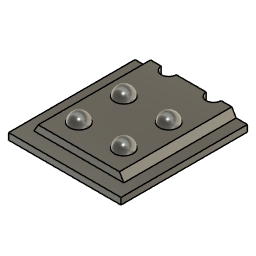
Rivets_Single riveted, single strap butt joint_Model (Autodesk Fusion 360 design; units mm, degrees)
Autodesk Fusion 360 part; units mm, degrees
note: some values were not read from the file. Set by a fixed rule: which sketch regions a step uses.
sketch "Sketch1" plane through (0, 0, 0) normal (0, 1, 0) x (1, 0, 0)
  line L0 (0, 0) -> (-60, 0)
  line L1 (-60, 0) -> (-60, 7)
  line L2 (-60, 7) -> (60, 7)
  line L3 (60, 7) -> (60, 0)
  line L4 (60, 0) -> (0, 0)
  line L5 (0, 0) -> (-48, 0)
  line L6 (0, 0) -> (48, 0)
  line L7 (0, 0) -> (0, -8)
  line L8 (0, -8) -> (-43.3812, -8)
  line L9 (-43.3812, -8) -> (0, -8)
  line L10 (0, -8) -> (43.3812, -8)
  line L11 (48, 0) -> (43.3812, -8)
  line L12 (48, 0) -> (78, 0) construction
  line L13 (-48, 0) -> (-43.3812, -8)
  line L14 (-48, 0) -> (-6.4505, 0) construction
  dimension "d1" = 60
  dimension "d2" = 7
  dimension "d3" = 120
  dimension "d4" = 7
  dimension "d5" = 48
  dimension "d6" = 48
  dimension "d7" = 8
  dimension "d9" = 120
  dimension "d11" = 60
  constraint coincident L0.start L4.end
  constraint horizontal L0
  constraint perpendicular L0 L1
  constraint perpendicular L1 L2
  constraint perpendicular L2 L3
  constraint perpendicular L3 L5
  constraint parallel L4 L6
  constraint perpendicular L6 L7
  constraint perpendicular L7 L8
  constraint perpendicular L7 L10
  constraint horizontal L12
  constraint horizontal L14
  measures "d1" distance of L0.start L0.end
  measures "d2" distance of L0.end L1.end
  measures "d3" distance of L1.end L2.end
  measures "d4" distance of L2.end L3.end
  measures "d5" distance of L0.start L5.end
  measures "d6" distance of L0.start L6.end
  measures "d7" distance of L0.start L7.end
  measures "d9" angle of L11 L12
  measures "d11" angle of L13 L14
extrude "Extrude1" add sketch "Sketch1" along normal mid plane 120 makes body 1
sketch "Sketch2" plane through (0, -60, 0) normal (0, -1, 0) x (1, 0, 0)
  line L0 (-48, 0) -> (-60, 0)
  line L1 (-60, 0) -> (-60, -7)
  line L2 (-60, -7) -> (60, -7)
  line L3 (60, -7) -> (60, 0)
  line L4 (60, 0) -> (48, 0)
  line L5 (48, 0) -> (43.3812, 8)
  line L6 (43.3812, 8) -> (-43.3812, 8)
  line L7 (-43.3812, 8) -> (-48, 0)
  line L8 (-48, 0) -> (48, 0)
  line L9 (48, 0) -> (60, 0)
  line L10 (60, 0) -> (60, -7)
  line L11 (60, -7) -> (-60, -7)
  line L12 (-60, -7) -> (-60, 0)
  line L13 (-60, 0) -> (-48, 0)
  constraint coincident L0.start L7.end
  constraint coincident L4.end L5.start
  constraint coincident L3.end L4.start
  constraint coincident L2.end L3.start
  constraint coincident L1.end L2.start
  constraint coincident L0.end L1.start
extrude "Extrude2" add sketch "Sketch2" along normal blind 15 contours L0 L1 L2 L3 L4 L8 L9 L10 L11 L12 L13 bodies 1
sketch "Sketch3" plane through (0, 0, 8) normal (0, 0, 1) x (-1, 0, 0)
  line L0 (-43.3812, 60) -> (-43.3812, -60)
  line L1 (-43.3812, -60) -> (43.3812, -60)
  line L2 (43.3812, -60) -> (43.3812, 60)
  line L3 (43.3812, 60) -> (-43.3812, 60)
  line L4 (0, -60) -> (0, 60)
  line L5 (0, -60) -> (24, -60)
  line L6 (24, 60) -> (-24, 60)
  circle A0 centre (-24, -60) radius 8
  circle A1 centre (24, -60) radius 8
  circle A2 centre (24, -12) radius 8
  circle A3 centre (24, 36) radius 8
  circle A4 centre (-24, -12) radius 8
  circle A5 centre (-24, 36) radius 8
  dimension "d16" = 24
  dimension "d17" = 24
  dimension "d18" = 48
  dimension "d19" = 16
  dimension "d20" = 16
  dimension "d21" = 48
  dimension "d22" = 16
  dimension "d23" = 48
  dimension "d24" = 16
  dimension "d25" = 48
  dimension "d26" = 16
  dimension "d27" = 48
  dimension "d28" = 16
  constraint midpoint L1 L4.start
  constraint midpoint L3 L4.end
  constraint perpendicular L4 L5
  constraint coincident L3 L6.start
  constraint perpendicular L4 L6
  constraint coincident L5.end A1.centre
  measures "d16" distance of L4.start A0.centre
  measures "d17" distance of L4.start L5.end
  measures "d18" distance of L6.start L6.end
  measures "d19" diameter of A0
  measures "d20" diameter of A1
  measures "d21" distance of L5.end A2.centre
  measures "d22" diameter of A2
  measures "d23" distance of A2.centre A3.centre
  measures "d24" diameter of A3
  measures "d25" distance of A0.centre A4.centre
  measures "d26" diameter of A4
  measures "d27" distance of A4.centre A5.centre
  measures "d28" diameter of A5
extrude "Extrude3" cut sketch "Sketch3" against normal blind 300 contours L1 A0 | L1 A0 | L1 L5 A1 | L1 L5 A1 | A2 | A3 | A4 | A5 bodies 1
sketch "Sketch4" plane through (0, 60, 0) normal (0, 1, 0) x (-1, 0, 0)
  line L0 (-32, -7) -> (-32, 8)
  line L1 (-32, 8) -> (-43.3812, 8)
  line L2 (-43.3812, 8) -> (-48, 0)
  line L3 (-48, 0) -> (-60, 0)
  line L4 (-60, 0) -> (-60, -7)
  line L5 (-60, -7) -> (-32, -7)
  line L6 (-133.6111, 10.5171) -> (-133.6111, -4.4829)
  line L7 (-133.6111, -4.4829) -> (-125.6111, -4.4829)
  line L8 (-125.6111, -4.4829) -> (-125.6111, 10.5171)
  line L9 (-125.6111, 10.5171) -> (-133.6111, 10.5171)
  line L10 (-133.6111, 10.5171) -> (-123.6111, 10.5171)
  line L11 (-133.6111, 10.5171) -> (-133.6111, 20.5171)
  line L12 (-133.6111, 10.5171) -> (-123.6111, 10.5171) construction
  line L13 (-133.6111, -4.4829) -> (-133.6111, -14.4829)
  line L14 (-133.6111, -4.4829) -> (-123.6111, -4.4829)
  line L15 (-133.6111, -4.4829) -> (-123.6111, -4.4829) construction
  arc A0 (-123.6111, 10.5171) -> (-133.6111, 20.5171) centre (-133.6111, 10.5171) ccw
  arc A1 (-133.6111, -14.4829) -> (-123.6111, -4.4829) centre (-133.6111, -4.4829) ccw
  dimension "d31" = 15
  dimension "d32" = 8
  dimension "d33" = 15
  dimension "d34" = 10
  dimension "d35" = 10
  dimension "d38" = 10
  dimension "d39" = 10
  constraint vertical L6
  constraint perpendicular L6 L7
  constraint perpendicular L7 L8
  constraint perpendicular L6 L10
  constraint perpendicular L10 L11
  constraint horizontal L12
  constraint perpendicular L7 L13
  constraint perpendicular L6 L14
  constraint horizontal L15
  measures "d31" distance of L6.start L6.end
  measures "d32" distance of L6.end L7.end
  measures "d33" distance of L7.end L8.end
  measures "d34" distance of L6.start L10.end
  measures "d35" distance of L6.start L11.end
  measures "d38" distance of L6.end L13.end
  measures "d39" distance of L6.end L14.end
revolve "Revolve1" add sketch "Sketch4" angle 360 about axis through (133.6111, 60, 10.5171) along (0, 0, -1) separate body contours L6 L7 L8 L9 L10 L14 | L9 L10 L11 A0 | L7 L13 L14 A1 makes body 2
copy_body "CopyPasteBodies1" bodies 2 makes body 3
move_body "Move1" bodies 3 to x (1, 0, 0) y (0, 1, 0) z (0, 0, 1) at (-109.6111, -48, -2.5171)
copy_body "CopyPasteBodies2" bodies 2 makes body 4
move_body "Move2" bodies 4 to x (1, 0, 0) y (0, 1, 0) z (0, 0, 1) at (-157.6111, -48, -2.5171)
copy_body "CopyPasteBodies3" bodies 2 makes body 5
move_body "Move3" bodies 5 to x (1, 0, 0) y (0, 1, 0) z (0, 0, 1) at (-109.6111, -96, -2.5171)
move_body "Move4" bodies 2 to x (1, 0, 0) y (0, 1, 0) z (0, 0, 1) at (-157.6111, -96, -2.5171)
